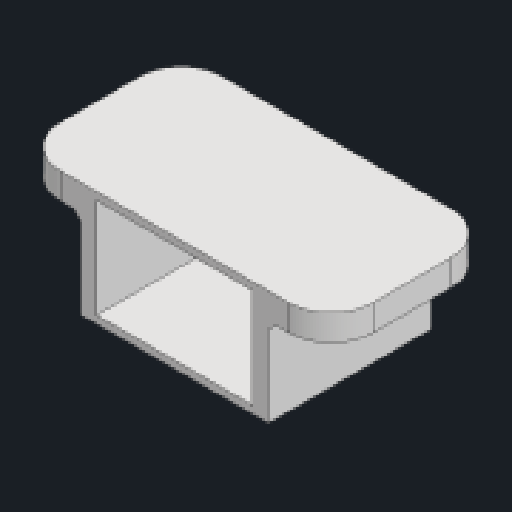
# Autodesk Inventor part: new_power_switch
Saved by Autodesk Inventor 2026 (Build 300175050, 175E)
## iProperties
Created: 2025-06-01
Part Number: new_power_switch
Material: Generic
Document SubType Name: Modeling
Designer: Natha
Density: 1 g/cm^3
Appearance: Default
Author: Natha
Autodesk Inventor part; units mm, degrees
ref_plane "YZ Plane" through (0, 0, 0) normal (1, 0, 0) x (0, 1, 0)
ref_plane "XZ Plane" through (0, 0, 0) normal (0, 1, 0) x (-1, 0, 0)
ref_plane "XY Plane" through (0, 0, 0) normal (0, 0, 1) x (1, 0, 0)
sketch "Sketch1" plane through (0, 0, 0) normal (0, 0, 1) x (1, 0, 0)
  ellipse E0 centre (0, 0) end of major axis (0, 70) minor radius 61.5 construction
  line L0 (-6.6, -55) -> (6.6, -55) construction
  line L1 (6.6, -55) -> (6.6, -63.55) construction
  line L2 (6.6, -63.55) -> (-6.6, -63.55) construction
  line L3 (-6.6, -63.55) -> (-6.6, -55) construction
  line L4 (0, 0) -> (0, -55) construction
  line L5 (-6.75, -54.5) -> (6.75, -54.5)
  line L6 (6.75, -54.5) -> (6.75, -64.05)
  line L7 (6.75, -64.05) -> (-6.75, -64.05)
  line L8 (-6.75, -64.05) -> (-6.75, -54.5)
  line L9 (9, -53.775) -> (-9, -53.775)
  line L10 (-9, -53.775) -> (-9, -64.775)
  line L11 (-9, -64.775) -> (9, -64.775)
  line L12 (9, -64.775) -> (9, -53.775)
  line L13 (6.75, -59.275) -> (-6.75, -59.275) construction
  line L14 (9, -53.775) -> (15, -53.775)
  line L15 (15, -53.775) -> (15, -56.275)
  line L16 (15, -56.275) -> (9, -56.275)
  line L17 (9, -56.275) -> (9, -53.775)
  line L18 (-9, -53.775) -> (-15, -53.775)
  line L19 (-15, -53.775) -> (-15, -56.275)
  line L20 (-15, -56.275) -> (-9, -56.275)
  dimension "d0" = 8.55
  dimension "d1" = 13.2
  dimension "d2" = 55
  dimension "d3" = 0.5
  dimension "d4" = 0.5
  dimension "d5" = 13.5
  dimension "d6" = 6.75
  dimension "d7" = 18
  dimension "d8" = 9
  dimension "d9" = 11
  dimension "d10" = 5.5
  dimension "d20" = 2.5
  dimension "d21" = 6
  constraints: 42 end point, 8 parallel, 4 horizontal, 4 perpendicular, 3 midpoint, 3 symmetric about line, 1 vertical, 1 other
  measures "d0" distance of L2.end L0.start
  measures "d1" distance of L1.end L2.end
  measures "d2" distance of L4.start L4.end
  measures "d3" distance between parallel lines of L7 L2
  measures "d4" distance between parallel lines of L5 L0
  measures "d5" distance of L6.end L7.end
  measures "d6" distance between parallel lines of L4 L8
  measures "d7" distance of L11.end L10.end
  measures "d8" distance between parallel lines of L12 L4
  measures "d9" distance of L11.end L9.start
  measures "d10" distance between parallel lines of L11 L13
  measures "d20" distance of L14.end L15.end
  measures "d21" distance of L9.start L14.end
extrude "Extrusion1" add sketch "Sketch1" against normal blind 15.6
sketch "Sketch2" plane through (0, 0, 0) normal (0, 0, 1) x (1, 0, 0)
  line L0 (-9, -56.275) -> (-9, -64.775) projected
  line L1 (-9, -64.775) -> (9, -64.775) projected
  line L2 (9, -64.775) -> (9, -56.275) projected
  line L3 (-6.75, -54.5) -> (6.75, -54.5) projected
  line L4 (6.75, -54.5) -> (6.75, -64.05) projected
  line L5 (6.75, -64.05) -> (-6.75, -64.05) projected
  line L6 (-6.75, -64.05) -> (-6.75, -54.5) projected
  line L7 (6.75, -54.5) -> (7.5, -54.5)
  line L8 (7.5, -54.5) -> (7.5, -64.05)
  line L9 (7.5, -64.05) -> (6.75, -64.05)
  line L10 (6.75, -64.05) -> (6.75, -54.5)
  line L11 (-6.75, -54.5) -> (-7.5, -54.5)
  line L12 (-7.5, -54.5) -> (-7.5, -64.05)
  line L13 (-7.5, -64.05) -> (-6.75, -64.05)
  line L14 (-6.75, -64.05) -> (-6.75, -54.5)
  line L15 (6.75, -64.05) -> (-6.75, -64.05) projected
  line L16 (9, -56.275) -> (15, -56.275) projected
  line L17 (15, -56.275) -> (15, -53.775) projected
  line L18 (15, -53.775) -> (-15, -53.775) projected
  line L19 (-15, -53.775) -> (-15, -56.275) projected
  line L20 (-15, -56.275) -> (-9, -56.275) projected
  point P0 (0, 0)
  dimension "d13" = 0.75
  dimension "d14" = 0.75
  constraints: 16 end point, 4 parallel, 2 collinear, 2 horizontal, 2 perpendicular, 1 point on line
  measures "d13" distance of L12.end L13.end
  measures "d14" distance of L8.end L9.end
extrude "Extrusion2" cut sketch "Sketch2" against normal blind 13.6 contours L6 L13 L12 L11 | L7 L8 L9 L4
chamfer "Chamfer1" distance 0.75 angle 45 2 edges at (7.5, -59.275, -13.6) (-7.5, -59.275, -13.6)
fillet "Fillet1" radius 4 4 edges at (15, -55.025, -15.6) (15, -55.025, 0) (-15, -55.025, 0) (-15, -55.025, -15.6)
chamfer "Chamfer2" distance 0.75 angle 45 2 edges at (9, -56.275, -7.8) (-9, -56.275, -7.8)
equation "\"d6\" = 0.5 * d5"
equation "\"d8\" = 0.5 * d7"
equation "\"d10\" = 0.5 * d9"
body "Solid1"
